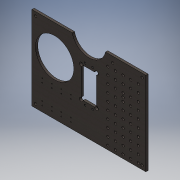
# Autodesk Inventor part: A0001
Saved by Autodesk Inventor 2017 (Build 210142000, 142)
## iProperties
Part Number: A0001
Material: ABS 塑膠
Document SubType Name: Modeling
Designer: lygfy
Density: 1.06 g/cm^3
Appearance: 胡桃木
Author: lygfy
Autodesk Inventor part; units mm, degrees
ref_plane "YZ Plane" through (0, 0, 0) normal (1, 0, 0) x (0, 1, 0)
ref_plane "XZ Plane" through (0, 0, 0) normal (0, 1, 0) x (-1, 0, 0)
ref_plane "XY Plane" through (0, 0, 0) normal (0, 0, 1) x (1, 0, 0)
sketch "草圖1" plane through (0, 0, 0) normal (0, 1, 0) x (-1, 0, 0)
  line L0 (7.5, -20) -> (-7.5, -20)
  line L1 (-10, -17.5) -> (-10, 17.5)
  line L2 (-7.5, 20) -> (7.5, 20)
  line L3 (10, 17.5) -> (10, -17.5)
  line L4 (75, 50) -> (75, -60)
  line L5 (75, -60) -> (-75, -60)
  line L6 (-75, -60) -> (-75, 50)
  arc A0 (-7.5, 20) -> (-10, 17.5) centre (-10, 20) ccw
  arc A1 (10, 17.5) -> (7.5, 20) centre (10, 20) ccw
  arc A2 (7.5, -20) -> (10, -17.5) centre (10, -20) ccw
  arc A3 (-10, -17.5) -> (-7.5, -20) centre (-10, -20) ccw
  arc A4 (-21.9374, 50) -> (21.9374, 50) centre (0, 55) ccw
  line L7 (-75, 50) -> (-21.9374, 50)
  line L8 (21.9374, 50) -> (75, 50)
  point P0 (0, 0)
  point P1 (-10, 0)
  point P2 (0, 20)
  point P3 (-10, 0)
  point P4 (0, -60)
  dimension "d2" = 5
  dimension "d3" = 40
  dimension "d4" = 20
  dimension "d19" = 45
  dimension "d20" = 55
  dimension "d21" = 150
  dimension "d30" = 110
  dimension "d31" = 60
  constraints: 18 end point, 10 point on circle, 8 point on line, 5 centre point, 4 midpoint, 3 equal radius, 3 horizontal, 3 parallel, 3 vertical alignment, 2 horizontal alignment, 2 vertical, 1 collinear, 1 perpendicular
  measures "d2" diameter of A0
  measures "d3" distance between parallel lines of L0 L2
  measures "d4" distance between parallel lines of L1 L3
  measures "d19" diameter of A4
  measures "d20" distance of point (0, 0) A4.centre
  measures "d21" distance of L4.end L5.end
  measures "d30" distance of L4.start L4.end
  measures "d31" distance from line of L5 point (0, 0)
extrude "擠出1" add sketch "草圖1" along normal mid plane 3
sketch "草圖4" plane through (0, -1.5, 0) normal (0, -1, 0) x (1, 0, 0)
  line L0 (-70, 45) -> (70, 45)
  line L1 (70, 45) -> (70, -55)
  line L2 (70, -55) -> (-70, -55)
  line L3 (-70, -55) -> (-70, 45)
  line L4 (75, -60) -> (75, 50) projected
  line L5 (-21.9374, 50) -> (-75, 50) projected
  point P0 (0, 0)
  point P1 (0, -55)
  dimension "d32" = 5
  dimension "d34" = 5
  dimension "d35" = 5
  constraints: 8 end point, 2 parallel, 1 horizontal, 1 midpoint, 1 perpendicular, 1 vertical alignment
  measures "d32" distance between parallel lines of L1 L4
  measures "d34" distance between parallel lines of L0 L5
  measures "d35" distance from line of L4.start L2
hole "孔3" at (-70, -1.5, 45) at (-70, -1.5, -55) at (70, -1.5, 45) at (70, -1.5, -55) direction (0, 1, 0) diameter 3.2 end through all
sketch "草圖2" plane through (0, -1.5, 0) normal (0, -1, 0) x (1, 0, 0)
  line L0 (-5, 24) -> (5, 24)
  line L1 (5, 24) -> (5, -24)
  line L2 (5, -24) -> (-5, -24)
  line L3 (-5, -24) -> (-5, 24)
  point P0 (0, 0)
  point P1 (5, 0)
  point P2 (0, 24)
  dimension "d9" = 10
  dimension "d10" = 48
  constraints: 8 end point, 2 midpoint, 2 parallel, 1 horizontal, 1 horizontal alignment, 1 perpendicular, 1 vertical alignment
  measures "d9" distance of L1.end L2.end
  measures "d10" distance of L0.end L1.end
hole "孔1" at (-5, -1.5, 24) at (5, -1.5, 24) at (5, -1.5, -24) at (-5, -1.5, -24) direction (0, 1, 0) diameter 2.459 depth 8.8 tip angle 118 thread size "M3x0.5" class "6H" standard "ISO Metric profile"
sketch "草圖3" plane through (0, -1.5, 0) normal (0, -1, 0) x (1, 0, 0)
  arc A0 (0, 77.5) -> (0, 32.5) centre (0, 55) ccw projected
  point P0 (45, 10)
  point P1 (31.3889, 42.245)
hole "孔2" at (31.3889, -1.5, 42.245) at (45, -1.5, 10) direction (0, 1, 0) diameter 3.2 end through all
sketch "草圖5" plane through (0, -1.5, 0) normal (0, -1, 0) x (1, 0, 0)
  circle A0 centre (-45, 10) radius 25.25
  point P0 (0, 0)
  dimension "d84" = 45
  dimension "d85" = 10
  dimension "d86" = 50.5
  constraints: 1 centre point
  measures "d84" horizontal distance of point (0, 0) A0.centre
  measures "d85" vertical distance of point (0, 0) A0.centre
  measures "d86" diameter of A0
extrude "擠出2" cut sketch "草圖5" along normal through all both and the other way through all
sketch "草圖6" plane through (0, 0, 0) normal (0, 1, 0) x (-1, 0, 0)
  line L0 (98, 0) -> (-98, 0) construction
  line L1 (0, -82) -> (0, 72) construction
  circle A0 centre (-25, -55) radius 1.6
  circle A1 centre (-25, -45) radius 1.6
  circle A2 centre (-25, -35) radius 1.6
  circle A3 centre (-25, -25) radius 1.6
  circle A4 centre (-25, -15) radius 1.6
  circle A5 centre (-35, -55) radius 1.6
  circle A6 centre (-35, -45) radius 1.6
  circle A7 centre (-35, -35) radius 1.6
  circle A8 centre (-35, -25) radius 1.6
  circle A9 centre (-35, -15) radius 1.6
  circle A10 centre (-45, -55) radius 1.6
  circle A11 centre (-45, -45) radius 1.6
  circle A12 centre (-45, -35) radius 1.6
  circle A13 centre (-45, -25) radius 1.6
  circle A14 centre (-45, -15) radius 1.6
  circle A15 centre (-55, -55) radius 1.6
  circle A16 centre (-55, -45) radius 1.6
  circle A17 centre (-55, -35) radius 1.6
  circle A18 centre (-55, -25) radius 1.6
  circle A19 centre (-55, -15) radius 1.6
  circle A20 centre (-65, -55) radius 1.6
  circle A21 centre (-65, -45) radius 1.6
  circle A22 centre (-65, -35) radius 1.6
  circle A23 centre (-65, -25) radius 1.6
  circle A24 centre (-65, -15) radius 1.6
  circle A25 centre (-25, -5) radius 1.6
  circle A26 centre (-35, -5) radius 1.6
  circle A27 centre (-45, -5) radius 1.6
  circle A28 centre (-55, -5) radius 1.6
  circle A29 centre (-65, -5) radius 1.6
  circle A30 centre (-25, 5) radius 1.6
  circle A31 centre (-35, 5) radius 1.6
  circle A32 centre (-45, 5) radius 1.6
  circle A33 centre (-55, 5) radius 1.6
  circle A34 centre (-65, 5) radius 1.6
  circle A35 centre (-25, 15) radius 1.6
  circle A36 centre (-35, 15) radius 1.6
  circle A37 centre (-45, 15) radius 1.6
  circle A38 centre (-55, 15) radius 1.6
  circle A39 centre (-65, 15) radius 1.6
  circle A40 centre (-25, 25) radius 1.6
  circle A41 centre (-35, 25) radius 1.6
  circle A42 centre (-45, 25) radius 1.6
  circle A43 centre (-55, 25) radius 1.6
  circle A44 centre (-65, 25) radius 1.6
  circle A45 centre (-25, 35) radius 1.6
  circle A46 centre (-35, 35) radius 1.6
  circle A47 centre (-45, 35) radius 1.6
  circle A48 centre (-55, 35) radius 1.6
  circle A49 centre (-65, 35) radius 1.6
  line L2 (75, 50) -> (75, -60) projected
  line L3 (75, -60) -> (-75, -60) projected
  line L4 (-75, -60) -> (-75, 50) projected
  circle A50 centre (61.25, -52.5) radius 0.6
  circle A51 centre (48.75, -52.5) radius 0.6
  circle A52 centre (61.25, -47.5) radius 0.6
  circle A53 centre (48.75, -47.5) radius 0.6
  line L5 (61, -56) -> (49, -56) construction
  line L6 (49, -56) -> (49, -44) construction
  line L7 (49, -44) -> (61, -44) construction
  line L8 (61, -44) -> (61, -56) construction
  line L9 (61, -56) -> (49, -44) construction
  line L10 (49, -56) -> (61, -44) construction
  line L11 (61.25, -52.5) -> (48.75, -47.5) construction
  line L12 (48.75, -52.5) -> (61.25, -47.5) construction
  circle A54 centre (36.25, -52.5) radius 0.6
  circle A55 centre (23.75, -52.5) radius 0.6
  circle A56 centre (23.75, -47.5) radius 0.6
  circle A57 centre (36.25, -47.5) radius 0.6
  circle A58 centre (61.25, -26.5) radius 0.6
  circle A59 centre (48.75, -26.5) radius 0.6
  circle A60 centre (48.75, -21.5) radius 0.6
  circle A61 centre (61.25, -21.5) radius 0.6
  circle A62 centre (36.25, -26.5) radius 0.6
  circle A63 centre (23.75, -26.5) radius 0.6
  circle A64 centre (23.75, -21.5) radius 0.6
  circle A65 centre (36.25, -21.5) radius 0.6
  point P0 (0, 0)
  point P1 (55, -50)
  dimension "d54" = 3.2
  dimension "d57" = 10
  dimension "d60" = 10
  dimension "d67" = 5
  dimension "d68" = 50
  dimension "d69" = 1.2
  dimension "d70" = 12.5
  dimension "d71" = 5
  dimension "d72" = 12
  dimension "d73" = 12
  dimension "d74" = 20
  dimension "d75" = 10
  dimension "d78" = 25
  dimension "d81" = 26
  constraints: 66 centre point, 16 end point, 3 equal radius, 3 horizontal, 2 horizontal alignment, 2 midpoint, 2 parallel, 2 vertical, 2 vertical alignment, 1 perpendicular, 122 other
  measures "d54" diameter of A0
  measures "d57" distance of A0.centre A1.centre
  measures "d60" distance of A0.centre A5.centre
  measures "d67" distance from line of A0.centre L3
  measures "d68" distance from line of L4 A0.centre
  measures "d69" diameter of A50
  measures "d70" distance of L12.start L11.start
  measures "d71" distance of L12.end L11.start
  measures "d72" distance of L6.end L7.end
  measures "d73" distance of L5.end L6.end
  measures "d74" distance from line of point (55, -50) L2
  measures "d75" distance from line of L3 point (55, -50)
  measures "d78" distance of L11.start A54.centre
  measures "d81" distance of L11.start A58.centre
extrude "擠出3" cut sketch "草圖6" along normal through all both and the other way through all
equation "\"d34\" = d33"
equation "\"d35\" = d32"
equation "\"d33\" = 5"
